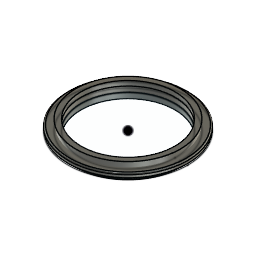
crank-pulley-centering-ring (Autodesk Fusion 360 design; units mm, degrees)
part number: 2026-05-14-22-13-22-884
Autodesk Fusion 360 part; units mm, degrees
sketch "inner and outer rings of pulley" plane through (0, 0, 0) normal (0, 0, 1) x (1, 0, 0)
  circle A0 centre (0, 0) radius 25.96
  circle A1 centre (0, 0) radius 32.98
  circle A2 centre (0, 0) radius 28.885
  dimension "d1" = 51.92
  dimension "d5" = 65.96
  dimension "d12" = 57.77
  constraint coincident A0.centre A1.centre
  constraint concentric A1 A2
  measures "d1" diameter of A0
  measures "d5" diameter of A1
  measures "d12" diameter of A2
extrude "Extrude1" add sketch "inner and outer rings of pulley" along normal blind 2.993 contours A1 | A2 makes body 1
extrude "Extrude2" add sketch "inner and outer rings of pulley" along normal blind -3.07 and the other way blind -5.633 separate body contours A2 makes body 2
fillet "Fillet4" radius 0.75 2 edges at (-30.7482, -11.9261, 2.993) (-30.7482, -11.9261, 0) on bodies 1
fillet "Fillet1" [suppressed]
fillet "Fillet2" [suppressed]
named bodies: "outer ring", "inner ring"
